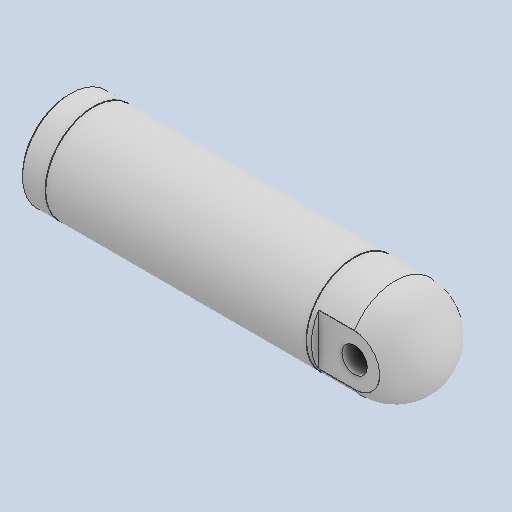
# Autodesk Inventor part: ANT-38-Body
Saved by Autodesk Inventor 2025.2 (Build 292293000, 293)
## iProperties
Created: 2026-01-25
Part Number: ANT-38-Body
Material: Generic
Document SubType Name: Modeling
Designer: LattePanda
Density: 1 g/cm^3
Appearance: Default
Author: LattePanda
Autodesk Inventor part; units mm, degrees
sketch "Body" plane through (0, 0, 0) normal (0, 1, 0) x (-1, 0, 0)
  circle A0 centre (0, 0) radius 5
  circle A1 centre (0, 0) radius 19
  line L0 (0, -19) -> (128.5, -19)
  line L1 (128.5, -19) -> (128.5, 19)
  line L2 (128.5, 19) -> (0, 19)
  line L3 (0, 19) -> (0, -19)
  line L4 (158, 0) -> (-48.5, 0) construction
  line L5 (0, -26.6) -> (0, 26.6) construction
  line L6 (-19, 0) -> (128.5, 0)
  point P0 (0, 0)
  dimension "d0" = 10
  dimension "d1" = 38
  dimension "d2" = 38
  dimension "d3" = 128.5
  constraints: 10 end point, 3 point on line, 2 centre point, 2 coincident, 2 midpoint, 2 parallel, 2 point on circle, 1 horizontal, 1 perpendicular
  measures "d0" diameter of A0
  measures "d1" diameter of A1
  measures "d2" distance of L2.end L0.start
  measures "d3" distance between parallel lines of L1 L3
revolve "BodyFeature" add sketch "Body" angle 360 about axis through (19, 0, 0) along (-1, 0, 0) picked at (14.1328, -1.7802) picked at (1.7623, -2.8047) picked at (-1.7802, -14.1328) picked at (-0.3709, -3.2915) contours L6 A1 L3 A0 | A0 L3 L6 | L3 A1 L6 A0 | A0 L6 L3 | L6 L1 L0 A1
ref_plane "Work Plane1" through (0, 0, -16) normal (0, 0, 1) x (1, 0, 0)
ref_plane "Work Plane2" through (0, 0, 16) normal (0, 0, 1) x (1, 0, 0)
sketch "Sketch2" plane through (0, 0, -16) normal (0, 0, 1) x (1, 0, 0)
  arc A0 (0, -19) -> (0, 19) centre (0, 0) ccw projected
  arc A1 (0, -10) -> (0, 10) centre (0, 0) ccw
  line L0 (0, -19) -> (0, -10) construction
  line L1 (0, 19) -> (0, -19) construction
  line L2 (0, -10) -> (-14, -10)
  line L3 (-14, -10) -> (-14, 10)
  line L4 (-14, 10) -> (0, 10)
  line L5 (-14, 10) -> (-14, -10)
  dimension "d7" = 10
  dimension "d8" = 14
  constraints: 10 end point, 2 point on circle, 1 centre point, 1 collinear, 1 horizontal, 1 parallel, 1 perpendicular, 1 point on line
  measures "d7" radius of A1
  measures "d8" distance between parallel lines of L1 L3
extrude "Extrusion1" cut sketch "Sketch2" against normal through all
mirror "Mirror1" about plane through (0, 0, 0) normal (0, 0, 1) of "Extrusion1"
sketch "Sketch3" plane through (0, 0, -16) normal (0, 0, -1) x (-1, 0, 0)
  circle A0 centre (0, 0) radius 5
  dimension "d11" = 10
  constraints: 1 centre point, 1 coincident
  measures "d11" diameter of A0
extrude "Extrusion2" cut sketch "Sketch3" against normal through all
fillet "Fillet1" radius 1 1 edges at (-14, 0, -16)
ref_plane "Work Plane3" through (-16, 0, 0) normal (1, 0, 0) x (0, 1, 0)
sketch "Sketch4" plane through (-16, 0, 0) normal (1, 0, 0) x (0, 1, 0)
  circle A0 centre (0, 0) radius 19 projected
  circle A1 centre (0, 0) radius 18.75
  dimension "d16" = 0.25
  constraints: 1 centre point
  measures "d16" radial gap between concentric circles of A0 A1
extrude "Extrusion3" cut sketch "Sketch4" along normal mid plane 0.25
ref_plane "Work Plane4" through (-118.5, 0, 0) normal (-1, 0, 0) x (0, 0, 1)
sketch "Sketch5" plane through (-118.5, 0, 0) normal (-1, 0, 0) x (0, 0, 1)
  circle A0 centre (0, 0) radius 19 projected
  circle A1 centre (0, 0) radius 18.75
  dimension "d20" = 0.25
  constraints: 1 centre point
  measures "d20" radial gap between concentric circles of A0 A1
extrude "Extrusion4" cut sketch "Sketch5" along normal mid plane 0.25
chamfer "Chamfer1" distance 1 angle 45 1 edges at (-128.5, 0, 19)
body "Solid1"
